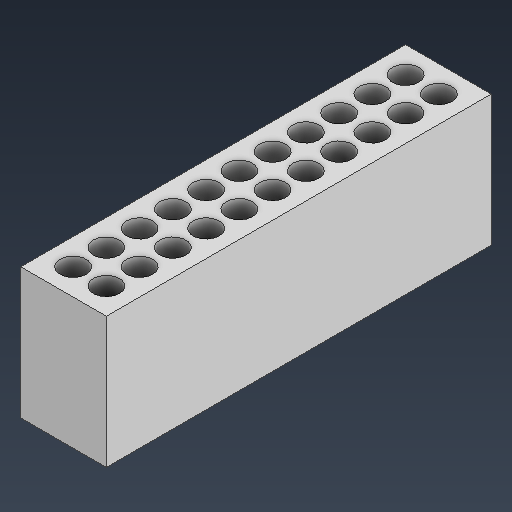
# Autodesk Inventor part: Button Header Spacer
Saved by Autodesk Inventor 2025.3 (Build 293356000, 356)
## iProperties
Created: 2025-09-24
Part Number: Button Header Spacer
Material: Generic
Document SubType Name: Modeling
Designer: tolga
Density: 1 g/cm^3
Appearance: Default
Author: tolga
Autodesk Inventor part; units mm, degrees
ref_plane "YZ Plane" through (0, 0, 0) normal (1, 0, 0) x (0, 1, 0)
ref_plane "XZ Plane" through (0, 0, 0) normal (0, 1, 0) x (-1, 0, 0)
ref_plane "XY Plane" through (0, 0, 0) normal (0, 0, 1) x (1, 0, 0)
sketch "Sketch1" plane through (0, 0, 0) normal (0, 1, 0) x (-1, 0, 0)
  circle A0 centre (0, 0) radius 1
  line L0 (2, 2) -> (-4.54, 2)
  line L1 (-4.54, 2) -> (-4.54, -27.4)
  line L2 (-4.54, -27.4) -> (2, -27.4)
  line L3 (2, -27.4) -> (2, 2)
  circle A1 centre (-2.54, 0) radius 1
  circle A2 centre (0, -2.54) radius 1
  circle A3 centre (-2.54, -2.54) radius 1
  circle A4 centre (0, -5.08) radius 1
  circle A5 centre (-2.54, -5.08) radius 1
  circle A6 centre (0, -7.62) radius 1
  circle A7 centre (-2.54, -7.62) radius 1
  circle A8 centre (0, -10.16) radius 1
  circle A9 centre (-2.54, -10.16) radius 1
  circle A10 centre (0, -12.7) radius 1
  circle A11 centre (-2.54, -12.7) radius 1
  circle A12 centre (0, -15.24) radius 1
  circle A13 centre (-2.54, -15.24) radius 1
  circle A14 centre (0, -17.78) radius 1
  circle A15 centre (-2.54, -17.78) radius 1
  circle A16 centre (0, -20.32) radius 1
  circle A17 centre (-2.54, -20.32) radius 1
  circle A18 centre (0, -22.86) radius 1
  circle A19 centre (-2.54, -22.86) radius 1
  circle A20 centre (0, -25.4) radius 1
  circle A21 centre (-2.54, -25.4) radius 1
  dimension "d0" = 2
  dimension "d3" = 2.54
  dimension "d6" = 2.54
  dimension "d9" = 1
  dimension "d10" = 1
  dimension "d11" = 1
  dimension "d12" = 1
  constraints: 22 centre point, 8 end point, 2 horizontal, 2 parallel, 1 coincident, 1 perpendicular, 1 vertical, 42 other
  measures "d0" diameter of A0
  measures "d3" distance of A0.centre A1.centre
  measures "d6" distance of A0.centre A2.centre
  measures "d9" distance edge to line of A10 L3
  measures "d10" distance edge to line of A11 L1
  measures "d11" distance edge to line of A1 L0
  measures "d12" distance edge to line of A20 L2
extrude "Extrusion1" add sketch "Sketch1" along normal blind 10
body "Solid1"
